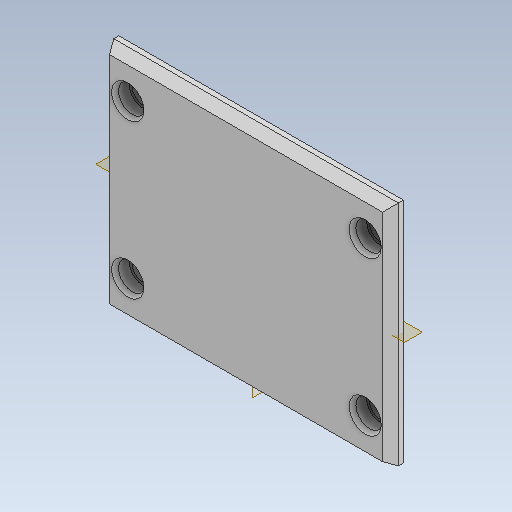
# Autodesk Inventor part: крышка
Saved by Autodesk Inventor 2021 (Build 250183000, 183)
## iProperties
Created: 2024-05-10
Part Number: крышка
Material: Типовые
Document SubType Name: Modeling
Designer: Мария
Density: 1 g/cm^3
Appearance: По умолчанию
Mass: 4.01868 g
Surface Area: 54.5848 cm^2
Volume: 4.01868 cm^3
Author: Мария
Autodesk Inventor part; units mm, degrees
ref_plane "YZ Plane" through (0, 0, 0) normal (1, 0, 0) x (0, 1, 0)
ref_plane "XZ Plane" through (0, 0, 0) normal (0, 1, 0) x (-1, 0, 0)
ref_plane "XY Plane" through (0, 0, 0) normal (0, 0, 1) x (1, 0, 0)
sketch "Эскиз1" plane through (0, 0, 0) normal (0, 0, 1) x (1, 0, 0)
  line L0 (0, 0) -> (52.9, 0)
  line L1 (52.9, 0) -> (52.9, 41.6)
  line L2 (52.9, 41.6) -> (0, 41.6)
  line L3 (0, 41.6) -> (0, 0)
  line L4 (0.2, 39.395) -> (52.7, 39.395) construction
  line L5 (0.2, 1.395) -> (0.2, 39.395) construction
  point P0 (6.0487, 0)
  point P1 (52.9, 1.3461)
  dimension "d0" = 38
  dimension "d1" = 52.5
  dimension "d2" = 41.6
  dimension "d3" = 52.9
  constraints: 8 end point, 2 parallel, 1 horizontal, 1 perpendicular
  measures "d0" distance of L5.start L4.start
  measures "d1" distance of L4.start L4.end
  measures "d2" distance of L2.end L0.start
  measures "d3" distance of L1.end L2.end
extrude "Выдавливание1" add sketch "Эскиз1" along normal blind 1.6
sketch "Эскиз2" plane through (0, 0, 1.6) normal (0, 0, 1) x (1, 0, 0)
  line L0 (-1.8, 43.4) -> (54.7, 43.4)
  line L1 (54.7, 43.4) -> (54.7, -1.8)
  line L2 (54.7, -1.8) -> (-1.8, -1.8)
  line L3 (-1.8, -1.8) -> (-1.8, 43.4)
  line L4 (0, 41.6) -> (0, 0) construction
  line L5 (52.9, 41.6) -> (0, 41.6) construction
  line L6 (52.9, 0) -> (52.9, 41.6) construction
  line L7 (0, 0) -> (52.9, 0) construction
  line L8 (1.8, 39.8) -> (51.1, 39.8)
  line L9 (51.1, 39.8) -> (51.1, 1.8)
  line L10 (51.1, 1.8) -> (1.8, 1.8)
  line L11 (1.8, 1.8) -> (1.8, 39.8)
  point P0 (52.9, 1.3461)
  point P1 (6.0487, 0)
  dimension "d6" = 1.8
  dimension "d7" = 1.8
  dimension "d8" = 1.8
  dimension "d9" = 1.8
  dimension "d10" = 1.8
  dimension "d11" = 1.8
  dimension "d13" = 1.8
  dimension "d14" = 1.8
  constraints: 16 end point, 4 parallel, 2 horizontal, 2 perpendicular
  measures "d6" distance between parallel lines of L3 L4
  measures "d7" distance between parallel lines of L0 L5
  measures "d8" distance between parallel lines of L6 L1
  measures "d9" distance between parallel lines of L7 L2
  measures "d10" distance between parallel lines of L5 L8
  measures "d11" distance between parallel lines of L4 L11
  measures "d13" distance between parallel lines of L9 L6
  measures "d14" distance between parallel lines of L7 L10
extrude "Выдавливание2" add sketch "Эскиз2" along normal blind 3 contours L0 L1 L2 L3 | L8 L9 L10 L11
ref_plane "РабПлоскость1" through (-1.8, 20.8, 1.6) normal (0, 1, 0) x (1, 0, 0)
ref_plane "РабПлоскость2" through (26.45, -1.8, 1.6) normal (1, 0, 0) x (0, 0, -1)
sketch "Эскиз3" plane through (0, 0, 4.6) normal (0, 0, 1) x (1, 0, 0)
  circle A0 centre (25.83, 5.555) radius 1.651 projected
  circle A1 centre (2.97, 5.555) radius 1.651 projected
  circle A2 centre (2.97, 36.035) radius 1.651 projected
  circle A3 centre (25.83, 36.035) radius 1.651 projected
  circle A4 centre (50.1, 36.04) radius 1.25 projected
  circle A5 centre (50.1, 5.56) radius 1.25 projected
  circle A6 centre (50.1, 5.56) radius 1.651
  circle A7 centre (50.1, 36.04) radius 1.651
  point P0 (0, 0)
  dimension "d30" = 3.302
  dimension "d31" = 3.302
  dimension "d32" = 3.302
  constraints: 2 centre point, 2 coincident
  measures "d30" diameter of A0
  measures "d31" diameter of A6
  measures "d32" diameter of A7
extrude "Выдавливание3" cut sketch "Эскиз3" against normal through all contours A1 | A2 | A4 | A5 | A6 | A7
sketch "Эскиз4" plane through (0, 0, 4.6) normal (0, 0, 1) x (1, 0, 0)
  line L0 (-1.8, -1.8) -> (54.7, -1.8) projected
  line L1 (54.7, -1.8) -> (54.7, 43.4) projected
  line L2 (54.7, 43.4) -> (-1.8, 43.4) projected
  line L3 (-1.8, 43.4) -> (-1.8, -1.8) projected
  circle A0 centre (2.97, 5.555) radius 2.7
  circle A1 centre (2.97, 36.035) radius 2.7
  circle A2 centre (50.1, 5.56) radius 2.7
  circle A3 centre (50.1, 36.04) radius 2.7
  circle A4 centre (50.1, 36.04) radius 1.651 projected
  circle A5 centre (50.1, 5.56) radius 1.651 projected
  circle A6 centre (25.83, 36.035) radius 1.651 projected
  circle A7 centre (2.97, 36.035) radius 1.651 projected
  circle A8 centre (25.83, 5.555) radius 1.651 projected
  circle A9 centre (2.97, 5.555) radius 1.651 projected
  circle A10 centre (25.83, 36.035) radius 2.7
  circle A11 centre (25.83, 5.555) radius 2.7
  point P0 (0, 0)
  dimension "d25" = 5.4
  dimension "d26" = 5.4
  dimension "d27" = 5.4
  dimension "d28" = 5.4
  dimension "d33" = 5.4
  dimension "d34" = 5.4
  constraints: 6 centre point, 6 coincident
  measures "d25" diameter of A0
  measures "d26" diameter of A1
  measures "d27" diameter of A2
  measures "d28" diameter of A3
  measures "d33" diameter of A10
  measures "d34" diameter of A11
extrude "Выдавливание4" cut sketch "Эскиз4" against normal blind 3 contours A0 | A1 | A2 | A3 | A4 | A5 | A7 | A9
chamfer "Фаска1" distance 1.1547 angle 60 4 edges at (-1.8, 20.8, 4.6) (26.45, 43.4, 4.6) (26.45, -1.8, 4.6) (54.7, 20.8, 4.6) measured on face at (-1.3, 20.8, 4.6) measured on face at (54.2, 20.8, 4.6) measured on face at (26.45, -1.3, 4.6) measured on face at (26.45, 42.9, 4.6)
sketch "Эскиз5" plane through (0, 0, 0) normal (0, 0, -1) x (-1, 0, 0)
  line L0 (-6.22, 1.6) -> (-46.85, 1.6)
  line L1 (-51.3, 8.81) -> (-51.3, 32.79)
  line L2 (-46.85, 40) -> (-6.22, 40)
  line L3 (-1.6, 32.785) -> (-1.6, 8.805)
  line L4 (0, 0) -> (-52.9, 0) projected
  line L5 (0, 41.6) -> (0, 0) projected
  line L6 (-52.9, 0) -> (-52.9, 41.6) projected
  line L7 (-52.9, 41.6) -> (0, 41.6) projected
  circle A0 centre (-2.97, 5.555) radius 1.651 projected
  arc A1 (-2.97, 8.805) -> (-6.22, 5.555) centre (-2.97, 5.555) ccw
  line L8 (-6.22, 5.555) -> (-6.22, 1.6)
  line L9 (-2.97, 8.805) -> (-1.6, 8.805)
  circle A2 centre (-2.97, 36.035) radius 1.651 projected
  arc A3 (-6.22, 36.035) -> (-2.97, 32.785) centre (-2.97, 36.035) ccw
  circle A4 centre (-50.1, 36.04) radius 1.651 projected
  circle A5 centre (-50.1, 5.56) radius 1.651 projected
  arc A6 (-50.1, 32.79) -> (-46.85, 36.04) centre (-50.1, 36.04) ccw
  arc A7 (-46.85, 5.56) -> (-50.1, 8.81) centre (-50.1, 5.56) ccw
  line L10 (-46.85, 36.04) -> (-46.85, 40)
  line L11 (-50.1, 8.81) -> (-51.3, 8.81)
  line L12 (-46.85, 5.56) -> (-46.85, 1.6)
  line L13 (-50.1, 32.79) -> (-51.3, 32.79)
  line L14 (-6.22, 36.035) -> (-6.22, 40)
  line L15 (-2.97, 32.785) -> (-1.6, 32.785)
  dimension "d38" = 1.6
  dimension "d39" = 1.6
  dimension "d40" = 1.6
  dimension "d41" = 1.6
  dimension "d42" = 6.5
  dimension "d43" = 6.5
  dimension "d44" = 6.5
  dimension "d45" = 6.5
  constraints: 24 end point, 9 perpendicular, 8 point on circle, 6 tangent, 4 centre point, 4 coincident, 2 parallel, 1 horizontal, 1 horizontal alignment, 1 vertical alignment
  measures "d38" distance between parallel lines of L4 L0
  measures "d39" distance between parallel lines of L5 L3
  measures "d40" distance between parallel lines of L6 L1
  measures "d41" distance between parallel lines of L2 L7
  measures "d42" diameter of A1
  measures "d43" diameter of A3
  measures "d44" diameter of A6
  measures "d45" diameter of A7
extrude "Выдавливание5" cut sketch "Эскиз5" against normal blind 2 contours L0 L12 A7 L11 L1 L13 A6 L10 L2 L14 A3 L15 L3 L9 A1 L8
sketch "Эскиз6" plane through (-1.8, -1.8, 1.6) normal (-1, 0, 0) x (0, 0, 1)
  line L0 (-17.4, 0) -> (0, 0) projected
  line L1 (0, 12.5304) -> (0, 0) projected
  line L2 (0, 12.5304) -> (-3.93, 12.5304) projected
  arc A0 (-3.93, 17.9304) -> (-3.93, 12.5304) centre (-3.93, 15.2304) ccw projected
  line L3 (-3.93, 17.9304) -> (0, 17.9304) projected
  line L4 (0, 45.2) -> (0, 17.9304) projected
  line L5 (-17.4, 45.2) -> (0, 45.2) projected
  line L6 (-1.63, 18.2304) -> (-1.63, 15.2304) projected
  line L7 (-1.63, 15.2304) -> (-1.63, 12.2304) projected
  line L8 (0, 17.7304) -> (-1.43, 17.7304)
  line L9 (-1.43, 17.7304) -> (-1.43, 12.7304)
  line L10 (-1.43, 12.7304) -> (0, 12.7304)
  line L11 (0, 12.7304) -> (0, 17.7304)
  line L12 (-17.4, 0) -> (-17.4, 45.2) projected
  point P0 (-1.6, 1.8)
  dimension "d48" = 0.2
  dimension "d49" = 0.2
  dimension "d50" = 0.2
  constraints: 8 end point, 2 parallel, 1 horizontal, 1 perpendicular, 1 vertical alignment
  measures "d48" distance between parallel lines of L2 L10
  measures "d49" distance between parallel lines of L8 L3
  measures "d50" distance between parallel lines of L6 L9
extrude "Выдавливание6" add sketch "Эскиз6" against normal up to surface (1.8 mm away) contours L11 L10 L9 L8
chamfer "Фаска2" distance 0.5 angle 60 1 edges at (1.319, 36.035, 1.6) measured on face at (0.819, 36.035, 1.6)
chamfer "Фаска3" distance 0.5 angle 60 1 edges at (1.319, 5.555, 1.6) measured on face at (0.819, 5.555, 1.6)
chamfer "Фаска4" distance 0.5 angle 60 1 edges at (48.449, 36.04, 1.6) measured on face at (47.949, 36.04, 1.6)
chamfer "Фаска5" distance 0.5 angle 60 1 edges at (48.449, 5.56, 1.6) measured on face at (47.949, 5.56, 1.6)
chamfer "Фаска6" distance 0.5 angle 60 4 edges at (0.27, 5.555, 4.6) (0.27, 36.035, 4.6) (47.4, 36.04, 4.6) (47.4, 5.56, 4.6) measured on face at (46.9, 36.04, 4.6) measured on face at (-0.23, 5.555, 4.6) measured on face at (46.9, 5.56, 4.6) measured on face at (-0.23, 36.035, 4.6)
equation "\"d7\" = d6"
equation "\"d8\" = d6"
equation "\"d9\" = d6"
equation "\"d10\" = d6"
equation "\"d11\" = d6"
equation "\"d13\" = d6"
equation "\"d14\" = d6"
equation "\"d31\" = d30"
equation "\"d32\" = d31"
equation "\"d26\" = d25"
equation "\"d27\" = d25"
equation "\"d28\" = d25"
equation "\"d33\" = d28"
equation "\"d34\" = d27"
